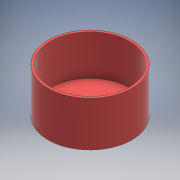
# Autodesk Inventor part: Jacket for wheel
Saved by Autodesk Inventor 2018 (Build 220112000, 112)
## iProperties
Created: 2019-03-26
Part Number: Jacket for wheel
Material: Типовые
Document SubType Name: Modeling
Designer: cosko
Density: 1 g/cm^3
Appearance: По умолчанию
Author: cosko
Autodesk Inventor part; units mm, degrees
ref_plane "YZ Plane" through (0, 0, 0) normal (1, 0, 0) x (0, 1, 0)
ref_plane "XZ Plane" through (0, 0, 0) normal (0, 1, 0) x (-1, 0, 0)
ref_plane "XY Plane" through (0, 0, 0) normal (0, 0, 1) x (1, 0, 0)
sketch "Эскиз1" plane through (0, 0, 0) normal (0, 0, 1) x (1, 0, 0)
  circle A0 centre (0, 0) radius 25 construction
  circle A1 centre (0, 0) radius 2.5
  circle A2 centre (0, 0) radius 26.5
  circle A3 centre (0, 0) radius 28
  dimension "d0" = 50
  dimension "d1" = 5
  dimension "d2" = 53
  dimension "d3" = 56
  constraints: 4 centre point, 4 coincident
  measures "d0" diameter of A0
  measures "d1" diameter of A1
  measures "d2" diameter of A2
  measures "d3" diameter of A3
extrude "Выдавливание1" add sketch "Эскиз1" along normal blind 3 contours A2
extrude "Выдавливание2" add sketch "Эскиз1" along normal blind 30 contours A3
